Mirror (Autodesk Fusion 360 design; units mm, degrees)
Autodesk Fusion 360 part; units mm, degrees
sketch "Sketch1" plane through (0, 0, 0) normal (0, 1, 0) x (1, 0, 0) in component "Servo"
  line L0 (0, 0) -> (28.5, 0)
  line L1 (28.5, 0) -> (28.5, -22.5)
  line L2 (28.5, -22.5) -> (0, -22.5)
  line L3 (0, -22.5) -> (0, 0)
  line L4 (18.05, -22.5) -> (20.5, -22.5)
  line L5 (20.5, -22.5) -> (20.5, -27.7)
  line L6 (20.5, -27.7) -> (18.05, -27.7)
  line L7 (18.05, -27.7) -> (18.05, -22.5)
  line L8 (18.05, 5.2) -> (20.5, 5.2)
  line L9 (20.5, 5.2) -> (20.5, 0)
  line L10 (20.5, 0) -> (18.05, 0)
  line L11 (18.05, 0) -> (18.05, 5.2)
  dimension "d1" = 28.5
  dimension "d2" = 22.5
  dimension "d3" = 2.45
  dimension "d4" = 5.2
  dimension "d5" = 2.45
  dimension "d6" = 5.2
  dimension "d7" = 8
  dimension "d8" = 8
  constraint horizontal L0
  constraint vertical L1
  constraint horizontal L2
  constraint vertical L3
  constraint coincident L0.start L3.end
  constraint horizontal L4
  constraint vertical L5
  constraint horizontal L6
  constraint vertical L7
  constraint horizontal L8
  constraint vertical L9
  constraint horizontal L10
  constraint vertical L11
  constraint collinear L2 L4
  constraint collinear L0 L10
  measures "d1" distance of L0.start L0.end
  measures "d2" distance of L0.start L2.end
  measures "d3" distance of L4.start L4.end
  measures "d4" distance of L4.start L6.end
  measures "d5" distance of L8.start L8.end
  measures "d6" distance of L8.start L10.end
  measures "d7" distance of L1 L5
  measures "d8" distance of L1 L9
extrude "Extrude1" add sketch "Sketch1" along normal blind 12 makes body 1 in component "Servo"
sketch "Sketch2" plane through (28.5, 0, 0) normal (1, 0, 0) x (0, 1, 0) in component "Servo"
  line L0 (0, 22.5) -> (0, 0)
  line L1 (0, 0) -> (12, 0)
  line L2 (12, 0) -> (12, 22.5)
  line L3 (12, 22.5) -> (0, 22.5)
  circle A0 centre (6, 16.75) radius 3.5
  line L4 (3.5, 16.75) -> (8.5, 16.75)
  line L5 (8.5, 16.75) -> (8.5, 1.75)
  line L6 (8.5, 1.75) -> (3.5, 1.75)
  line L7 (3.5, 1.75) -> (3.5, 16.75)
  circle A1 centre (6, 3.75) radius 0.9
  dimension "d11" = 7
  dimension "d13" = 5.75
  dimension "d14" = 6
  dimension "d15" = 5
  dimension "d16" = 15
  dimension "d157" = 1.8
  dimension "d158" = 2.5
  dimension "d159" = 2
  constraint horizontal L4
  constraint vertical L5
  constraint horizontal L6
  constraint vertical L7
  constraint midpoint A0.centre L4
  measures "d11" diameter of A0
  measures "d13" distance of L3 A0.centre
  measures "d14" distance of L2 A0.centre
  measures "d15" distance of L4.start L4.end
  measures "d16" distance of L4.start L6.end
  measures "d157" diameter of A1
  measures "d158" distance of L5 A1.centre
  measures "d159" distance of L6 A1.centre
extrude "Extrude2" add sketch "Sketch2" along normal blind 5 separate body contours A0 L4 L5 L7 | A0 L4 L5 L7 makes body 2 in component "Servo"
extrude "Extrude3" add sketch "Sketch2" along normal blind 1.5 from surface at 3.5 contours A0 L5 L6 L7 bodies 2 in component "Servo"
sketch "Sketch3" plane through (20.5, 0, 0) normal (1, 0, 0) x (0, 1, 0) in component "Servo"
  line L0 (0, 27.7) -> (0, 22.5)
  line L1 (0, 22.5) -> (12, 22.5)
  line L2 (12, 22.5) -> (12, 27.7)
  line L3 (12, 27.7) -> (0, 27.7)
  circle A0 centre (5.75, 25.325) radius 1.375
  circle A1 centre (5.75, -2.825) radius 1.375
  line L4 (0, -5.2) -> (12, -5.2)
  line L5 (12, 0) -> (12, -5.2)
  circle A2 centre (5.75, 25.325) radius 0.85
  circle A3 centre (5.75, -2.825) radius 0.85
  dimension "d22" = 2.75
  dimension "d23" = 2.375
  dimension "d24" = 6.25
  dimension "d25" = 2.75
  dimension "d26" = 2.375
  dimension "d27" = 6.25
  dimension "d41" = 1.7
  dimension "d42" = 1.7
  constraint concentric A0 A2
  constraint concentric A1 A3
  measures "d22" diameter of A0
  measures "d23" distance of L3 A0.centre
  measures "d24" distance of L2 A0.centre
  measures "d25" diameter of A1
  measures "d26" distance of A1.centre L4
  measures "d27" distance of A1.centre L5
  measures "d41" diameter of A2
  measures "d42" diameter of A3
fillet "Fillet1" radius 2 2 edges at (32.75, 3.5, 1.75) (32.75, 8.5, 1.75) on bodies 2 in component "Servo"
sketch "Sketch2 (2)" plane through (0, 0, 0) normal (0, 1, 0) x (1, 0, 0) in component "Servo Clamp"
  line L0 (8.5, -29.2) -> (20.5, -29.2)
  line L1 (20.5, -29.2) -> (20.5, 6.7)
  line L2 (20.5, 6.7) -> (8.5, 6.7)
  line L3 (8.5, 6.7) -> (8.5, -29.2)
  line L4 (18.05, 5.2) -> (20.5, 5.2)
  line L5 (20.5, -27.7) -> (18.05, -27.7)
  line L6 (0, -22.5) -> (0, 0)
  point P0 (20.5, -22.5)
  dimension "d32" = 1.5
  dimension "d33" = 1.5
  dimension "d69" = 12
  constraint horizontal L0
  constraint vertical L1
  constraint horizontal L2
  constraint vertical L3
  constraint coincident L1 P0
  measures "d32" distance of L2 L4
  measures "d33" distance of L0 L5
  measures "d69" distance of L1 L3
extrude "Extrude1'" add sketch "Sketch2 (2)" along normal blind 14 and the other way blind 2 separate body makes body 3 in component "Servo Clamp"
copy_body "CopyPasteBodies1" bodies 1 makes body 4 in component "Servo Clamp"
offset_surface "SurfaceOffset1" offset 0.2 14 faces at (6.0167, 12, 7.5) (12.0333, 4, 22.5) (6.0167, 0, 7.5) (18.05, 8, 24.2333) (18.05, 4, -1.7333) (19.6833, 4, 27.7) (18.8667, 4, -5.2) (20.5, 8, 25.9667) (28.5, 4, 7.5) (25.8333, 4, 22.5) (23.1667, 4, 0) (0, 4, 15) (6.0167, 4, 0) (20.5, 4, -3.4667) on bodies 4 makes body 5 in component "Servo Clamp"
stitch "SurfaceStitch1" surfaces 5 tolerance 0.1 makes body 6 in component "Servo Clamp"
sketch "Sketch4" plane through (0, 0, 0) normal (-1, 0, 0) x (0, -1, 0) in component "Servo"
  line L0 (0, 0) -> (0, 22.5)
  line L1 (0, 22.5) -> (-12, 22.5)
  line L2 (-12, 22.5) -> (-12, 0)
  line L3 (-12, 0) -> (0, 0)
  line L4 (-8.75, 23.1924) -> (-3.25, 23.1924)
  line L5 (-3.25, 23.1924) -> (-3.25, 20.4924)
  line L6 (-3.25, 20.4924) -> (-8.75, 20.4924)
  line L7 (-8.75, 20.4924) -> (-8.75, 23.1924)
  dimension "d46" = 5.5
  dimension "d47" = 2.7
  dimension "d48" = 3.25
  constraint horizontal L4
  constraint vertical L5
  constraint horizontal L6
  constraint vertical L7
  measures "d46" distance of L4.start L4.end
  measures "d47" distance of L4.start L6.end
  measures "d48" distance of L2 L7
combine "Combine2" operation cut target body 3 tool bodies 6 in component "Servo Clamp"
extrude "Extrude6" cut sketch "Sketch3" against normal blind 7 from surface at -1.7 contours A2 | A3 bodies 3 in component "Servo Clamp"
sketch "Sketch5" plane through (8.5, 0, 0) normal (-1, 0, 0) x (0, -1, 0) in component "Servo Clamp"
  line L0 (0.2, -0.2) -> (-12.2, -0.2)
  line L1 (-12.2, -0.2) -> (-12.2, 22.7)
  line L2 (-12.2, 22.7) -> (0.2, 22.7)
  line L3 (0.2, 22.7) -> (0.2, -0.2)
  line L4 (2, 29.2) -> (-14, 29.2)
  line L5 (-14, 29.2) -> (-14, -6.7)
  line L6 (-14, -6.7) -> (2, -6.7)
  line L7 (2, -6.7) -> (2, 29.2)
  circle A0 centre (7, 11.25) radius 2.25
  circle A1 centre (7, 11.25) radius 0.825
  line L8 (0.2, 13.5) -> (7, 13.5)
  line L9 (7, 13.5) -> (7, 9)
  line L10 (7, 9) -> (0.2, 9)
  line L11 (0.2, 9) -> (0.2, 13.5)
  dimension "d70" = 4.5
  dimension "d71" = 1.65
  dimension "d72" = 17.95
  dimension "d73" = 5
  constraint concentric A0 A1
  constraint horizontal L8
  constraint vertical L9
  constraint horizontal L10
  constraint vertical L11
  constraint coincident L3 L8.start
  constraint coincident A0.centre L9
  constraint tangent A0 L8
  constraint tangent A0 L10
  measures "d70" diameter of A0
  measures "d71" diameter of A1
  measures "d72" distance of L4 A0.centre
  measures "d73" distance of L7 A0.centre
extrude "Extrude11" add sketch "Sketch5" against normal blind 20 contours L3 L7 L8 L10 L11 bodies 3 in component "Servo Clamp"
fillet "Fillet3" radius 10 2 edges at (20.5, -1.1, 9) (20.5, -1.1, 13.5) on bodies 3 in component "Servo Clamp"
extrude "Extrude9" add sketch "Sketch5" against normal blind 4 from surface at -16 contours L3 L7 L8 L10 L11 | L7 A0 L8 L10 | A0 A1 L9 | A0 A1 L9 bodies 3 in component "Servo Clamp"
extrude "Extrude10" add sketch "Sketch5" against normal blind 4 from surface at -8 contours L3 L7 L8 L10 L11 | L7 A0 L8 L10 | A0 A1 L9 | A0 A1 L9 bodies 3 in component "Servo Clamp"
extrude "Extrude14" add sketch "Sketch5" against normal blind 4 contours L7 A0 L8 L10 | A0 A1 L9 | A0 A1 L9 bodies 3 in component "Servo Clamp"
extrude "Extrude1''" add sketch "Sketch5" against normal blind 3.6 from surface at -4.2 separate body contours A0 A1 L9 | A0 A1 L9 makes body 7 in component "Rocker"
sketch "Sketch1 (2)" plane through (8.5, 0, 0) normal (-1, 0, 0) x (0, -1, 0) in component "Rocker"
  line L0 (7, 13.5) -> (10.5, 13.5)
  line L1 (10.5, 13.5) -> (10.5, 9)
  line L2 (10.5, 9) -> (7, 9)
  line L3 (7, 9) -> (7, 13.5)
  circle A0 centre (7, 11.25) radius 2.25
  circle A1 centre (7, 11.25) radius 0.825
  point P0 (7, 11.25)
  dimension "d82" = 3.5
  dimension "d262" = 1.65
  constraint horizontal L0
  constraint vertical L1
  constraint horizontal L2
  constraint vertical L3
  constraint coincident L3 P0
  constraint tangent L2 A0
  constraint tangent L0 A0
  constraint coincident P0 A0.centre
  measures "d82" distance of L1.end L2.end
  measures "d262" diameter of A1
extrude "Extrude2'" add sketch "Sketch1 (2)" against normal blind 3.6 from surface at -4.2 contours L0 L1 L2 A0 bodies 7 in component "Rocker"
sketch "Sketch2 (3)" plane through (0, -10.5, 0) normal (0, -1, 0) x (1, 0, 0) in component "Rocker"
  line L0 (-5.5, 35.25) -> (42.5, 35.25)
  line L1 (42.5, 35.25) -> (42.5, -12.75)
  line L2 (42.5, -12.75) -> (-5.5, -12.75)
  line L3 (-5.5, -12.75) -> (-5.5, 35.25)
  line L4 (-5.5, -12.75) -> (42.5, 35.25)
  line L5 (6, 23.75) -> (31, 23.75)
  line L6 (31, 23.75) -> (31, -1.25)
  line L7 (31, -1.25) -> (6, -1.25)
  line L8 (6, -1.25) -> (6, 23.75)
  line L9 (6, 23.75) -> (31, -1.25)
  line L10 (32, -1.25) -> (33.5, -1.25)
  line L11 (33.5, -1.25) -> (33.5, 5.75)
  line L12 (33.5, 5.75) -> (32, 5.75)
  line L13 (32, 5.75) -> (32, -1.25)
  line L14 (-6.5, 36.25) -> (43.5, 36.25)
  line L15 (43.5, 36.25) -> (43.5, -13.75)
  line L16 (43.5, -13.75) -> (-6.5, -13.75)
  line L17 (-6.5, -13.75) -> (-6.5, 36.25)
  line L18 (-6.5, 36.25) -> (43.5, -13.75)
  line L19 (16.5, 13.5) -> (20.5, 13.5)
  line L20 (20.5, 13.5) -> (20.5, 9)
  line L21 (20.5, 9) -> (16.5, 9)
  line L22 (16.5, 9) -> (16.5, 13.5)
  line L23 (16.5, 13.5) -> (20.5, 9)
  point P0 (18.5, 11.25)
  point P1 (18.5, 11.25)
  point P2 (18.5, 11.25)
  point P3 (18.5, 11.25)
  point P4 (18.5, 11.25)
  dimension "d86" = 48
  dimension "d87" = 48
  dimension "d88" = 25
  dimension "d89" = 25
  dimension "d169" = 1.5
  dimension "d173" = 7
  dimension "d214" = 50
  dimension "d215" = 50
  dimension "d260" = 11.5
  dimension "d261" = 9
  constraint horizontal L0
  constraint vertical L1
  constraint horizontal L2
  constraint vertical L3
  constraint midpoint L4 P4
  constraint coincident P4 P3
  constraint horizontal L5
  constraint vertical L6
  constraint horizontal L7
  constraint vertical L8
  constraint midpoint L9 P4
  constraint horizontal L10
  constraint vertical L11
  constraint horizontal L12
  constraint vertical L13
  constraint horizontal L14
  constraint vertical L15
  constraint horizontal L16
  constraint vertical L17
  constraint midpoint L18 P4
  constraint horizontal L19
  constraint vertical L20
  constraint horizontal L21
  constraint vertical L22
  constraint midpoint L23 P4
  measures "d86" distance of L0.start L0.end
  measures "d87" distance of L0.end L1.end
  measures "d88" distance of L5.start L5.end
  measures "d89" distance of L5.start L7.end
  measures "d169" distance of L11.end L12.end
  measures "d173" distance of L10.start L12.end
  measures "d214" distance of L14.start L14.end
  measures "d215" distance of L14.start L16.end
  measures "d260" distance of L2 L10
  measures "d261" distance of L1 L11
extrude "Extrude3'" add sketch "Sketch2 (3)" along normal blind 1.5 contours L4 L8 L9 L18 L22 | L4 L5 L9 L18 L19 L20 L22 | L4 L6 L9 L18 L20 | L4 L7 L9 L18 L20 L21 L22 | L9 L18 L22 L23 | L4 L9 L18 L22 | L4 L9 L18 L20 | L4 L19 L20 L23 | L4 L21 L22 L23 | L9 L18 L20 L23 bodies 7 in component "Rocker"
extrude "Extrude7" add sketch "Sketch1 (2)" against normal blind 3.6 from surface at -12.2 contours L3 A0 A1 | L0 L1 L2 A0 | L3 A0 A1 bodies 7 in component "Rocker"
extrude "Extrude1'''" add sketch "Sketch2 (3)" along normal blind 2 from surface at 1.5 separate body contours L3 L4 L8 L18 | L0 L4 L5 L18 | L1 L4 L6 L18 | L2 L4 L7 L18 | L4 L8 L9 L18 L22 | L4 L5 L9 L18 L19 L20 L22 | L4 L6 L9 L18 L20 | L4 L7 L9 L18 L20 L21 L22 | L9 L18 L22 L23 | L4 L9 L18 L22 | L4 L9 L18 L20 | L4 L19 L20 L23 | L4 L21 L22 L23 | L9 L18 L20 L23 | L10 L11 L12 L13 makes body 8 in component "Plate"
fillet "Fillet1'" radius 5 4 edges at (42.5, -13, 35.25) (-5.5, -13, 35.25) (42.5, -13, -12.75) (-5.5, -13, -12.75) on bodies 8 in component "Plate"
copy_body "Body->Comp1" bodies 2 removing the originals makes body 9 in component "Servo Arm"
extrude "Extrude4" add sketch "Sketch2 (3)" along normal blind 1.5 contours L3 L4 L8 L18 | L0 L4 L5 L18 | L1 L4 L6 L18 | L2 L4 L7 L18 | L4 L8 L9 L18 L22 | L4 L5 L9 L18 L19 L20 L22 | L4 L6 L9 L18 L20 | L4 L7 L9 L18 L20 L21 L22 | L9 L18 L22 L23 | L4 L9 L18 L22 | L4 L9 L18 L20 | L4 L19 L20 L23 | L4 L21 L22 L23 | L9 L18 L20 L23 | L10 L11 L12 L13 bodies 7 in component "Rocker"
extrude "Extrude5" add sketch "Sketch2 (3)" against normal blind 7 contours L10 L11 L12 L13 bodies 7 in component "Rocker"
sketch "Sketch3 (2)" plane through (33.5, 0, 0) normal (1, 0, 0) x (0, 1, 0) in component "Rocker"
  line L0 (-10.5, 5.75) -> (-10.5, -1.25)
  line L1 (-10.5, -1.25) -> (-3.5, -1.25)
  line L2 (-3.5, -1.25) -> (-3.5, 5.75)
  line L3 (-3.5, 5.75) -> (-10.5, 5.75)
  circle A0 centre (-7, 2.25) radius 0.9
  line L4 (-3.5, 5.75) -> (-10.5, -1.25)
  point P0 (-7, 2.25)
  point P1 (-7, 2.25)
  dimension "d130" = 1.8
  constraint coincident P1 P0
  constraint coincident L2.end L3.start
  constraint coincident L0.end L1.start
  constraint midpoint L4 P1
  measures "d130" diameter of A0
extrude "Extrude6'" cut sketch "Sketch3 (2)" against normal blind 2 contours A0 L4 | A0 L4 bodies 7 in component "Rocker"
fillet "Fillet2" radius 3.5 2 edges at (32.75, -3.5, 5.75) (32.75, -3.5, -1.25) on bodies 7 in component "Rocker"
sketch "Sketch1 (3)" plane through (33.4, 0, 0) normal (1, 0, 0) x (0, 1, 0) in component "Connector"
  circle A0 centre (-3.0091, 2.248) radius 0.9
  line L0 (-7.6603, 3.9409) -> (-4.702, -2.4032)
  arc A1 (-1.5299, -0.9241) -> (-4.4882, 5.4201) centre (-3.0091, 2.248) ccw
  line L1 (-8.8206, 8.6502) -> (7.1794, 8.6502)
  line L2 (7.1794, 8.6502) -> (7.1794, 3.6502)
  line L3 (7.1794, 3.6502) -> (-8.8206, 3.6502)
  line L4 (-8.8206, 3.6502) -> (-8.8206, 8.6502)
  circle A2 centre (-5.8206, 6.1502) radius 0.825
  circle A3 centre (4.1794, 6.1502) radius 0.825
  line L5 (-1.3206, 8.6502) -> (1.1794, 8.6502)
  line L6 (1.1794, 8.6502) -> (1.1794, 3.6502)
  line L7 (1.1794, 3.6502) -> (-1.3206, 3.6502)
  line L8 (-1.3206, 3.6502) -> (-1.3206, 8.6502)
  line L9 (-4.4882, 5.4201) -> (-7.6603, 3.9409)
  line L10 (-4.702, -2.4032) -> (-1.5299, -0.9241)
  dimension "d137" = 1.65
  dimension "d138" = 5
  dimension "d139" = 16
  dimension "d140" = 2.5
  dimension "d141" = 3
  dimension "d143" = 1.65
  dimension "d144" = 2.5
  dimension "d145" = 3
  dimension "d148" = 2.5
  dimension "d149" = 6
  constraint horizontal L1
  constraint vertical L2
  constraint horizontal L3
  constraint vertical L4
  constraint horizontal L5
  constraint vertical L6
  constraint horizontal L7
  constraint vertical L8
  constraint collinear L1 L5
  constraint collinear L3 L7
  measures "d137" diameter of A2
  measures "d138" distance of L1.start L3.end
  measures "d139" distance of L1.start L1.end
  measures "d140" distance of L1 A2.centre
  measures "d141" distance of L4 A2.centre
  measures "d143" diameter of A3
  measures "d144" distance of L1 A3.centre
  measures "d145" distance of L2 A3.centre
  measures "d148" distance of L5.start L5.end
  measures "d149" distance of L2 L6
extrude "Extrude1''''" add sketch "Sketch1 (3)" along normal blind 1.5 separate body contours L0 A1 L3 L8 L9 | L0 A1 L1 L3 L4 L8 L9 | A1 L3 L7 L8 | A1 L1 L3 L5 L6 L7 L8 | L1 L2 L3 L6 makes body 10 in component "Connector"
extrude "Extrude2''" add sketch "Sketch1 (3)" against normal blind 1.8 contours A1 L3 L7 L8 | A1 L1 L3 L5 L6 L7 L8 bodies 10 in component "Connector"
extrude "Extrude3''" add sketch "Sketch1 (3)" against normal blind 1.5 from surface at -1.8 contours L0 A1 L3 L8 L9 | L0 A1 L1 L3 L4 L8 L9 | A1 L3 L7 L8 | A1 L1 L3 L5 L6 L7 L8 | L1 L2 L3 L6 bodies 10 in component "Connector"
fillet "Fillet1''" radius 2 8 edges at (30.85, -8.8206, 8.6502) (34.15, -8.8206, 8.6502) (34.15, -8.8206, 3.6502) (30.85, -8.8206, 3.6502) (34.15, 7.1794, 8.6502) (30.85, 7.1794, 8.6502) (30.85, 7.1794, 3.6502) (34.15, 7.1794, 3.6502) on bodies 10 in component "Connector"
sketch "Sketch6" plane through (0, 14, 0) normal (0, 1, 0) x (-1, 0, 0) in component "Servo Clamp"
  line L0 (-8.5, -6.7) -> (-8.5, 29.2)
  line L1 (-8.5, 29.2) -> (-20.5, 29.2)
  line L2 (-20.5, 29.2) -> (-20.5, -6.7)
  line L3 (-20.5, -6.7) -> (-8.5, -6.7)
  line L4 (-30.0818, 24.35) -> (-28.4363, 21.5)
  line L5 (-28.4363, 21.5) -> (-25.1454, 21.5)
  line L6 (-25.1454, 21.5) -> (-23.5, 24.35)
  line L7 (-23.5, 24.35) -> (-25.1454, 27.2)
  line L8 (-25.1454, 27.2) -> (-28.4363, 27.2)
  line L9 (-28.4363, 27.2) -> (-30.0818, 24.35)
  line L10 (-20.5, 29.2) -> (-32.0818, 29.2)
  line L11 (-32.0818, 29.2) -> (-32.0818, 19.5)
  line L12 (-32.0818, 19.5) -> (-20.5, 19.5)
  line L13 (-20.5, 19.5) -> (-20.5, 29.2)
  circle A0 centre (-26.7909, 24.35) radius 1.5
  line L14 (-23.5, -1.85) -> (-25.1454, 1)
  line L15 (-32.0818, -6.7) -> (-20.5, -6.7)
  line L16 (-30.0818, -1.85) -> (-28.4363, -4.7)
  line L17 (-20.5, -6.7) -> (-20.5, 3)
  line L18 (-28.4363, 1) -> (-30.0818, -1.85)
  circle A1 centre (-26.7909, -1.85) radius 1.5
  line L19 (-32.0818, 3) -> (-32.0818, -6.7)
  line L20 (-25.1454, -4.7) -> (-23.5, -1.85)
  line L21 (-28.4363, -4.7) -> (-25.1454, -4.7)
  line L22 (-20.5, 3) -> (-32.0818, 3)
  line L23 (-25.1454, 1) -> (-28.4363, 1)
  line L24 (-20.5, 29.2) -> (-33.5818, 29.2)
  line L25 (-33.5818, 29.2) -> (-33.5818, 30.7)
  line L26 (-33.5818, 30.7) -> (-20.5, 30.7)
  line L27 (-20.5, 30.7) -> (-20.5, 29.2)
  line L28 (-32.0818, 19.5) -> (-33.5818, 19.5)
  line L29 (-33.5818, 19.5) -> (-33.5818, 29.2)
  line L30 (-33.5818, 29.2) -> (-32.0818, 29.2)
  line L31 (-32.0818, 29.2) -> (-32.0818, 19.5)
  line L32 (-32.0818, 3) -> (-33.5818, 3)
  line L33 (-33.5818, 3) -> (-33.5818, -8.2)
  line L34 (-33.5818, -8.2) -> (-32.0818, -8.2)
  line L35 (-32.0818, -8.2) -> (-32.0818, 3)
  line L36 (-20.5, -6.7) -> (-32.0818, -6.7)
  line L37 (-32.0818, -6.7) -> (-32.0818, -8.2)
  line L38 (-32.0818, -8.2) -> (-20.5, -8.2)
  line L39 (-20.5, -8.2) -> (-20.5, -6.7)
  point P0 (-26.7909, 24.35)
  point P1 (-20.5, 29.2)
  point P2 (-26.7909, -1.85)
  dimension "d191" = 2.85
  dimension "d192" = 2
  dimension "d193" = 2
  dimension "d194" = 2
  dimension "d195" = 3
  dimension "d196" = 3
  dimension "d203" = 2.85
  dimension "d204" = 2
  dimension "d205" = 2
  dimension "d206" = 2
  dimension "d207" = 3
  dimension "d208" = 3
  dimension "d223" = 1.5
  dimension "d224" = 1.5
  dimension "d225" = 1.5
  dimension "d226" = 1.5
  constraint horizontal L8
  constraint horizontal L10
  constraint vertical L11
  constraint horizontal L12
  constraint vertical L13
  constraint coincident P0 A0.centre
  constraint horizontal L23
  constraint horizontal L22
  constraint vertical L19
  constraint horizontal L15
  constraint vertical L17
  constraint coincident P2 A1.centre
  constraint coincident P1 L1.end
  constraint coincident L2.end L3.start
  constraint horizontal L24
  constraint vertical L25
  constraint horizontal L26
  constraint vertical L27
  constraint horizontal L28
  constraint vertical L29
  constraint horizontal L30
  constraint vertical L31
  constraint coincident L24 L25.start
  constraint coincident L24.end L25.start
  constraint horizontal L32
  constraint vertical L33
  constraint horizontal L34
  constraint vertical L35
  constraint horizontal L36
  constraint vertical L37
  constraint horizontal L38
  constraint vertical L39
  constraint coincident L35 L34.end
  constraint coincident L34.end L35.start
  measures "d191" distance of P0 L9
  measures "d192" distance of L8 L10
  measures "d193" distance of L5 L12
  measures "d194" distance of L4.start L11
  measures "d195" distance of L6.end L13
  measures "d196" diameter of A0
  measures "d203" distance of P2 L18
  measures "d204" distance of L22 L23
  measures "d205" distance of L15 L21
  measures "d206" distance of L16.start L19
  measures "d207" distance of L14.start L17
  measures "d208" diameter of A1
  measures "d223" distance of P1 L26.end
  measures "d224" distance of L11.end L28.end
  measures "d225" distance of L19.start L32.end
  measures "d226" distance of L2.end L38.end
extrude "Extrude12" add sketch "Sketch6" against normal blind 3 from surface at 1.2 contours L0 L1 L2 L3 L13 L17 | L2 L15 L17 L19 L22 L35 L36 | L2 L10 L11 L12 L13 L24 L31 | L4 L5 L6 L7 L8 L9 | L14 L16 L18 L20 L21 L23 bodies 3 in component "Servo Clamp"
extrude "Extrude13" cut sketch "Sketch6" against normal blind 5 from surface at -0.3 contours L4 L5 L6 L7 L8 L9 | L14 L16 L18 L20 L21 L23 bodies 3 in component "Servo Clamp"
fillet "Fillet4" radius 5 4 edges at (42.5, -11.25, 35.25) (-5.5, -11.25, 35.25) (-5.5, -11.25, -12.75) (42.5, -11.25, -12.75) on bodies 7 in component "Rocker"
extrude "Extrude2'''" [suppressed] in component "4by4 Grid"
extrude "Extrude3'''" [suppressed] in component "4by4 Grid"
extrude "Extrude5'" [suppressed] in component "4by4 Grid"
sketch "Sketch2 (4)" plane through (0, 15.7, 0) normal (0, -1, 0) x (1, 0, 0) in component "4by4 Grid"
  line L0 (24.5818, -8.2) -> (12.5, -8.2)
  line L1 (12.5, -8.2) -> (12.5, -6.7)
  line L2 (12.5, -6.7) -> (23.0818, -6.7)
  line L3 (23.0818, -6.7) -> (23.0818, 3)
  line L4 (23.0818, 3) -> (24.5818, 3)
  line L5 (24.5818, 3) -> (24.5818, -8.2)
  line L6 (23.0818, 19.5) -> (23.0818, 29.2)
  line L7 (23.0818, 29.2) -> (12.5, 29.2)
  line L8 (12.5, 29.2) -> (12.5, 30.7)
  line L9 (12.5, 30.7) -> (24.5818, 30.7)
  line L10 (24.5818, 30.7) -> (24.5818, 19.5)
  line L11 (24.5818, 19.5) -> (23.0818, 19.5)
  circle A0 centre (17.7909, 24.35) radius 1.5
  circle A1 centre (17.7909, -1.85) radius 1.5
  line L12 (-10.6, -13.75) -> (39.4, -13.75)
  line L13 (39.4, -13.75) -> (39.4, 36.25)
  line L14 (39.4, 36.25) -> (-10.6, 36.25)
  line L15 (-10.6, 36.25) -> (-10.6, -13.75)
  line L16 (-8.35, 33.75) -> (36.9, 33.75)
  line L17 (36.9, 33.75) -> (36.9, -11.25)
  line L18 (36.9, -11.25) -> (-8.35, -11.25)
  line L19 (-8.35, -11.25) -> (-8.35, 33.75)
  line L20 (-5.35, 33.75) -> (33.9, 33.75)
  line L21 (33.9, 33.75) -> (33.9, -11.25)
  line L22 (33.9, -11.25) -> (-5.35, -11.25)
  line L23 (-5.35, -11.25) -> (-5.35, 33.75)
  line L24 (-5.35, 19.5) -> (33.9, 19.5)
  line L25 (33.9, 19.5) -> (33.9, 3)
  line L26 (33.9, 3) -> (-5.35, 3)
  line L27 (-5.35, 3) -> (-5.35, 19.5)
  line L28 (11.4, 19.5) -> (17.4, 19.5)
  line L29 (17.4, 19.5) -> (17.4, 3)
  line L30 (17.4, 3) -> (11.4, 3)
  line L31 (11.4, 3) -> (11.4, 19.5)
  line L32 (39.4, -31.9235) -> (39.4, 67.3839) construction
  line L33 (-24.4336, -13.75) -> (68.025, -13.75) construction
  dimension "d229" = 2.5
  dimension "d230" = 2.25
  dimension "d231" = 2.5
  dimension "d232" = 2.5
  dimension "d234" = 3
  dimension "d236" = 3
  dimension "d239" = 6
  dimension "d240" = 22
  constraint horizontal L16
  constraint vertical L17
  constraint horizontal L18
  constraint vertical L19
  constraint horizontal L20
  constraint vertical L21
  constraint horizontal L22
  constraint vertical L23
  constraint horizontal L24
  constraint vertical L25
  constraint horizontal L26
  constraint vertical L27
  constraint coincident L21 L25.end
  constraint coincident L23 L24.start
  constraint coincident L4.end L26
  constraint coincident L6.start L24
  constraint collinear L16 L20
  constraint collinear L18 L22
  constraint horizontal L28
  constraint vertical L29
  constraint horizontal L30
  constraint vertical L31
  constraint coincident L26 L29.end
  constraint coincident L24 L28.start
  constraint perpendicular L14 L32
  constraint perpendicular L32 L33
  measures "d229" distance of L14 L16
  measures "d230" distance of L15 L19
  measures "d231" distance of L12 L18
  measures "d232" distance of L13 L17
  measures "d234" distance of L17 L21
  measures "d236" distance of L19 L23
  measures "d239" distance of L29.end L30.end
  measures "d240" distance of L15 L31
extrude "Extrude6''" [suppressed] in component "4by4 Grid"
copy_body "CopyPasteBodies1'" [suppressed] in component "4by4 Grid"
move_body "Move1" [suppressed] in component "4by4 Grid"
combine "Combine1" [suppressed] in component "4by4 Grid"
copy_body "CopyPasteBodies2" [suppressed] in component "4by4 Grid"
move_body "Move2" [suppressed] in component "4by4 Grid"
combine "Combine2'" [suppressed] in component "4by4 Grid"
extrude "Extrude1'''''" [suppressed] in component "Stamp"
fillet "Fillet1'''" [suppressed] in component "Stamp"
extrude "Extrude2''''" [suppressed] in component "Stamp"
extrude "Extrude3''''" [suppressed] in component "Stamp"
extrude "Extrude4'" [suppressed] in component "Stamp"
extrude "Extrude5''" [suppressed] in component "Stamp"
component "Servo" placed x (1, 0, 0) y (0, 1, 0) z (0, 0, 1) at (-8, 0, 0)
component "Rocker" placed x (1, 0, 0) y (0, 1, 0) z (0, 0, 1) at (-0.1, 0, 0)
component "Servo Clamp" placed x (1, 0, 0) y (0, 1, 0) z (0, 0, 1) at (-0.1, 0, 0)
component "Plate" placed x (1, 0, 0) y (0, 1, 0) z (0, 0, 1) at (-0.1, 0, 0)
component "Connector" placed x (1, 0, 0) y (0, 1, 0) z (0, 0, 1) at (0.3, -1.1794, -3.9002)
component "Servo Arm" placed x (1, 0, 0) y (0, 1, 0) z (0, 0, 1) at (0, 0, 0) in component "Servo"
hidden bodies 4
